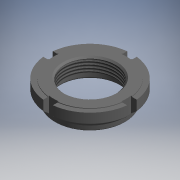
# Autodesk Inventor part: 1515746 GUA M28x1.5
Saved by Autodesk Inventor 2017.3 (Build 213256000, 256)
## iProperties
Part Number: 1515746 GUA M28x1.5
Material: Generic
Catalog Web Link: www.cadenas.de
Description: GUA-slotted round nut
Vendor: FESTO
Document SubType Name: Modeling
Designer: partserver
Manufacturer: FESTO
Mass: 7.91963 g
Surface Area: 40.5379 cm^2
Volume: 7.91963 cm^3
Density: 1 g/cm^3
Appearance: PSOLRGB-128-128-128
Category: PARTsolutions
Company: FESTO
Title: 1515746 GUA M28x1.5
Author: Cadenas PARTsolutions
Comments: slotted round nut
PSOL_IDENT_0: {$CADENAS_DATA\23d-libs\festo\parts\g\gua\gua.prj},175 {VTYP=3D},{NB=1515746 GUA M28x1.5},{LINA=1515
PSOL_IDENT_1: 746 GUA M28x1.5},{NN=GUA},{DATE=09.09.2015 14:14:39},{GEOMDATE=03.09.2015 07:34:17},{VERSION=},{LINE
PSOL_IDENT_2: ID=50},{WBVAR=},{WBNUMERIC=}  {NB=1515746 GUA M28x1.5},{LINA=1515746 GUA M28x1.5},{KT=DUMMY},{TNR=15
PSOL_IDENT_3: 15746},{TYP=GUA},{D=M28x1.5},{DN=28.000},{B=11.200},{B1=2.300},{D1=44.000},{D2=37.000},{A=39.000},{T=
PSOL_IDENT_4: 38.000},{C=5.000},{H=7.000},{P=1.500}
NB: 1515746 GUA M28x1.5
NN: GUA
NT: slotted round nut
NBSYN: $TNR. $TYP. $D.
LINA: 1515746 GUA M28x1.5
CATALOG: Festo
TNR: 1515746
TYP: GUA
D: M28x1.5
DN: 28
B: 11.2
B1: 2.3
D1: 44
D2: 37
A: 39
T: 38
C: 5
H: 7
P: 1.5
SUPPLIER: FESTO
ARTICLENO: 1515746 GUA M28x1.5
BOMINFO: 1515746 GUA M28x1.5
CREATOR: CADENAS GmbH
Autodesk Inventor part; units mm, degrees
sketch "Sketch_2" plane through (0, 0, 0) normal (1, 0, 0) x (0, 1, 0)
  line L0 (0, 0) -> (0, 11.2)
  line L1 (17.6596, 11.2) -> (16, 11.2)
  arc A0 (16, 11.2) -> (15, 10.2) centre (16, 10.2) ccw
  line L2 (15, 10.2) -> (15, 8.9)
  line L3 (15, 8.9) -> (14, 8.9)
  line L4 (14, 8.9) -> (14, 7)
  line L5 (14, 7) -> (13.188, 7)
  line L6 (13.188, 7) -> (13.188, 0.812)
  line L7 (13.188, 0.812) -> (14, 0)
  line L8 (14, 0) -> (19.5, 0)
  line L9 (19.5, 0) -> (19.5, 0.3)
  line L10 (19.5, 0.3) -> (22, 0.3)
  line L11 (22, 0.3) -> (22, 5.23)
  arc A1 (22, 5.23) -> (21.8214, 5.613) centre (21.5, 5.23) ccw
  line L12 (21.8214, 5.613) -> (18.7083, 8.2252)
  arc A2 (18.5316, 8.5646) -> (18.7083, 8.2252) centre (19.0297, 8.6082) ccw
  line L13 (18.5316, 8.5646) -> (18.357, 10.561)
  arc A3 (18.357, 10.561) -> (17.6596, 11.2) centre (17.6596, 10.5) ccw
  constraints: 28 end point, 8 point on circle, 4 centre point
revolve "Revolution1" add sketch "Sketch_2" angle 360 about axis through (0, 0, 0) along (0, 0, -1)
thread "Thread1" size "M28x1.5" class "6H" standard "ISO Metric profile" full length
sketch "Skizze_2" plane through (0, 0, 0) normal (0, 0, 1) x (1, 0, 0)
  line L0 (-44, 44) -> (-44, -44)
  line L1 (-44, -44) -> (44, -44)
  line L2 (44, -44) -> (44, 44)
  line L3 (44, 44) -> (-44, 44)
  arc A0 (-22.8637, -2.5) -> (-2.5, -22.8637) centre (0, 0) ccw
  line L4 (-2.5, -22.8637) -> (-2.5, -18.8348)
  arc A1 (-2.5, -18.8348) -> (2.5, -18.8348) centre (0, 0) ccw
  line L5 (2.5, -18.8348) -> (2.5, -22.8637)
  arc A2 (2.5, -22.8637) -> (22.8637, -2.5) centre (0, 0) ccw
  line L6 (22.8637, -2.5) -> (18.8348, -2.5)
  arc A3 (18.8348, -2.5) -> (18.8348, 2.5) centre (0, 0) ccw
  line L7 (18.8348, 2.5) -> (22.8637, 2.5)
  arc A4 (22.8637, 2.5) -> (2.5, 22.8637) centre (0, 0) ccw
  line L8 (2.5, 22.8637) -> (2.5, 18.8348)
  arc A5 (2.5, 18.8348) -> (-2.5, 18.8348) centre (0, 0) ccw
  line L9 (-2.5, 18.8348) -> (-2.5, 22.8637)
  arc A6 (-2.5, 22.8637) -> (-22.8637, 2.5) centre (0, 0) ccw
  line L10 (-22.8637, 2.5) -> (-18.8348, 2.5)
  arc A7 (-18.8348, 2.5) -> (-18.8348, -2.5) centre (0, 0) ccw
  line L11 (-18.8348, -2.5) -> (-22.8637, -2.5)
  constraints: 24 end point, 16 point on circle, 8 centre point
extrude "Extrusion1" cut sketch "Skizze_2" along normal blind 11.2
ref_plane "ANBAU_XY" through (0, 0, 0) normal (0, 0, 1) x (1, 0, 0)
ref_plane "ANBAU_YZ" through (0, 0, 0) normal (1, 0, 0) x (0, 1, 0)
ref_plane "ANBAU_ZX" through (0, 0, 0) normal (0, 1, 0) x (0, 0, 1)
body "Solid1"
